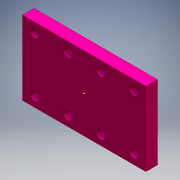
# Autodesk Inventor part: Coperchio
Saved by Autodesk Inventor 2016 (Build 200138000, 138)
## iProperties
Created: 2016-09-10
Part Number: Coperchio
Material: Generic
Document SubType Name: Modeling
Designer: Muhammad
Density: 1 g/cm^3
Appearance: Default
Author: Muhammad
Autodesk Inventor part; units mm, degrees
ref_plane "YZ Plane" through (0, 0, 0) normal (1, 0, 0) x (0, 1, 0)
ref_plane "XZ Plane" through (0, 0, 0) normal (0, 1, 0) x (-1, 0, 0)
ref_plane "XY Plane" through (0, 0, 0) normal (0, 0, 1) x (1, 0, 0)
sketch "Sketch1" plane through (0, 0, 0) normal (0, 1, 0) x (-1, 0, 0)
  point P0 (0, 0)
sketch "Sketch2" plane through (0, 0, 0) normal (0, 1, 0) x (-1, 0, 0)
  line L0 (-31.75, 19) -> (31.75, 19)
  line L1 (31.75, 19) -> (31.75, -19)
  line L2 (31.75, -19) -> (-31.75, -19)
  line L3 (-31.75, -19) -> (-31.75, 19)
  line L4 (-31.75, 19) -> (31.75, -19) construction
  line L5 (31.75, 19) -> (-31.75, -19) construction
  line L6 (31.75, 19) -> (25.5, 19) construction
  line L7 (-31.75, 19) -> (-31.75, 14) construction
  line L8 (-31.75, 14) -> (31.75, 14) construction
  line L9 (25.5, 19) -> (8.5, 19) construction
  line L10 (8.5, 19) -> (8.5, 14) construction
  line L11 (8.5, 19) -> (-8.5, 19) construction
  line L12 (-8.5, 19) -> (-8.5, 14) construction
  line L13 (-8.5, 19) -> (-25.5, 19) construction
  line L14 (-25.5, 19) -> (-25.5, 14) construction
  line L15 (31.75, 19) -> (25.5, 19) construction
  line L16 (25.5, 19) -> (25.5, 14) construction
  circle A0 centre (25.5, 14) radius 2.25
  circle A1 centre (8.5, 14) radius 2.25
  circle A2 centre (-8.5, 14) radius 2.25
  circle A3 centre (-25.5, 14) radius 2.25
  line L17 (31.75, 0) -> (-31.75, 0) construction
  circle A4 centre (25.5, -14) radius 2.25
  circle A5 centre (8.5, -14) radius 2.25
  circle A6 centre (-8.5, -14) radius 2.25
  circle A7 centre (-25.5, -14) radius 2.25
  point P0 (0, 0)
  dimension "d3" = 5
  dimension "d7" = 4.5
  dimension "d8" = 4.5
  dimension "d9" = 4.5
  constraints: 36 end point, 10 point on line, 8 centre point, 6 perpendicular, 4 coincident, 4 midpoint, 4 symmetric about line, 2 horizontal, 2 parallel, 4 other
  measures "d3" distance of L0.start L7.end
  measures "d7" diameter of A0
  measures "d8" diameter of A1
  measures "d9" diameter of A2
extrude "Extrusion1" add sketch "Sketch2" along normal blind 6
body "Solid1"
